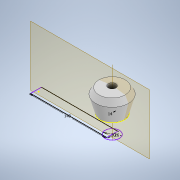
# Autodesk Inventor part: handle
Saved by Autodesk Inventor 2022 (Build 260153000, 153)
## iProperties
Created: 2021-03-11
Part Number: handle
Material: Generic
Document SubType Name: Modeling
Designer: ben
Density: 1 g/cm^3
Appearance: Default
Author: ben
Autodesk Inventor part; units mm, degrees
ref_plane "YZ Plane" through (0, 0, 0) normal (1, 0, 0) x (0, 1, 0)
ref_plane "XZ Plane" through (0, 0, 0) normal (0, 1, 0) x (-1, 0, 0)
ref_plane "XY Plane" through (0, 0, 0) normal (0, 0, 1) x (1, 0, 0)
sketch "Sketch1" plane through (0, 0, 0) normal (0, 0, 1) x (1, 0, 0)
  line L0 (5, -10) -> (-135, -10)
  line L1 (-135, -10) -> (-135, 10)
  line L2 (-135, 10) -> (5, 10)
  line L3 (5, 10) -> (5, -10)
  circle A0 centre (-135, 0) radius 13
  point P0 (0, 0)
  dimension "d0" = 140
  dimension "d1" = 20
  dimension "d5" = 26
  constraints: 8 end point, 2 parallel, 1 centre point, 1 horizontal, 1 horizontal alignment, 1 midpoint, 1 perpendicular
  measures "d0" distance of L1.end L2.end
  measures "d1" distance of L0.end L1.end
  measures "d5" diameter of A0
extrude "Extrusion1" add sketch "Sketch1" along normal blind 30 contours L0 A0 L2 L3 | L0 L1 L2 A0 picked at (-130.6667, 0)
fillet "Fillet1" radius 15 2 edges at (5, 0, 30) (5, 0, 0)
sketch "Sketch9" plane through (-10, 10, 15) normal (0, 1, 0) x (1, 0, 0)
  circle A0 centre (0, 0) radius 11.2
  point P0 (10, 15)
  dimension "d21" = 22.4
  constraints: 1 centre point
  measures "d21" diameter of A0
extrude "bearing hole 1" [suppressed]
ref_plane "Work Plane4" through (-10, 0, 15) normal (0, 1, 0) x (1, 0, 0)
sketch "Sketch19" plane through (-10, 0, 15) normal (0, 1, 0) x (1, 0, 0)
  circle A0 centre (0, 0) radius 11.2 projected
  circle A1 centre (0, 0) radius 4
  point P0 (10, 15)
  dimension "d59" = 8
  constraints: 1 centre point, 1 coincident
  measures "d59" diameter of A1
extrude "bearing hole 2" [suppressed]
sketch "Sketch23" plane through (-10, 0, 15) normal (0, 1, 0) x (1, 0, 0)
  line L0 (-103, -19) -> (-94.9615, -49)
  line L1 (-94.9615, -49) -> (-101.0237, -59.5)
  line L2 (-103, -19) -> (-118, -19)
  line L3 (-125, -15) -> (0, -15) projected
  line L4 (-125, -76.2) -> (-125, 30.2) projected
  line L5 (-118, -53.8801) -> (-118, -61.8801)
  line L6 (-118, -61.8801) -> (-101.0237, -59.5)
  line L7 (-118, -53.8801) -> (-118, -19)
  line L8 (-118, -53.8801) -> (-118, -53.8801)
  point P0 (10, 15)
  point P1 (-125, -19)
  dimension "d64" = 75
  dimension "d65" = 30
  dimension "d66" = 10.5
  dimension "d67" = 135
  dimension "d75" = 8
  dimension "d98" = 4
  dimension "d113" = 4
  dimension "d114" = 22
  dimension "d128" = 7
  dimension "d139" = 127.981
  dimension "d149" = 0
  constraints: 14 end point, 2 horizontal, 1 perpendicular, 1 point on line, 1 vertical, 1 other
  measures "d64" angle to the sketch x axis of L0
  measures "d65" vertical distance of L0.start L0.end
  measures "d66" vertical distance of L1.end L0.end
  measures "d67" angle of L0 L1
  measures "d75" distance of L5.start L5.end
  measures "d114" distance from line of L4 L0.start
  measures "d128" distance between parallel lines of L4 L7
  measures "d139" angle of L1 L6
  measures "d149" distance between parallel lines of L7 L5
sketch "Sketch26" plane through (-10, 0, 15) normal (0, 1, 0) x (1, 0, 0)
  line L0 (-138, 15) -> (-112, 15) projected
  line L1 (-125, 15) -> (-112, 15)
  line L2 (-125, -25.8) -> (-125, 21.8) projected
  line L3 (-125, 15) -> (0, 15) projected
  line L4 (-102.8897, -19) -> (-125, -19)
  line L5 (-125, -19) -> (-125, 15)
  line L6 (-112, 15) -> (-102.8897, -19)
  point P0 (10, 15)
  point P1 (-125, -15)
  dimension "d111" = 4
  dimension "d112" = 75
  constraints: 8 end point, 2 perpendicular, 1 collinear, 1 point on line
  measures "d111" distance of point (-125, -15) L4.end
  measures "d112" angle of L3 L6
revolve "Revolution2" add sketch "Sketch26" angle 360 about axis through (-135, 0, 30) along (0, 0, -1)
sketch "Sketch27" plane through (-135, 0, 34) normal (0, 0, 1) x (0, -1, 0)
  circle A0 centre (0, 0) radius 7
  circle A1 centre (0, 0) radius 22.1103 projected
  dimension "d79" = 14
  constraints: 1 centre point
  measures "d79" diameter of A0
extrude "Extrusion21" add sketch "Sketch27" along normal blind 34 contours A0
revolve "Revolution3" add sketch "Sketch23" angle 360 about axis through (-135, 0, 30) along (0, 0, -1) separate body
thicken "Thicken1" [suppressed]
thicken "Thicken2" [suppressed]
thicken "Thicken3" [suppressed]
thicken "Thicken4" [suppressed]
thicken "Thicken5" [suppressed]
sketch "Sketch32" plane through (-10, 10, 15) normal (0, 1, 0) x (1, 0, 0)
  circle A0 centre (0, 0) radius 4
  point P0 (10, 15)
  dimension "d125" = 8
  constraints: 1 centre point
  measures "d125" diameter of A0
extrude "simple bearing hole" cut sketch "Sketch32" against normal through all bodies 1
hole "Hole1" at (-135, 0, 68) direction (0, 0, -1) diameter 7 depth 20 tip angle 120 bodies 1
sketch "Sketch34" plane through (-135, 0, 68) normal (0, 0, 1) x (1, 0, 0)
  circle A0 centre (0, 0) radius 4
  circle A1 centre (0, 0) radius 3.5 projected
  circle A2 centre (0, 0) radius 7 projected
  circle A3 centre (0, 0) radius 6
  point P0 (135, 0)
  dimension "d145" = 8
  dimension "d148" = 12
  constraints: 2 centre point, 1 coincident
  measures "d145" diameter of A0
  measures "d148" diameter of A3
extrude "Extrusion27" cut sketch "Sketch34" against normal blind 6 bodies 1
